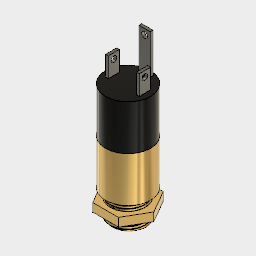
3692 TRS Jack (Autodesk Fusion 360 design; units mm, degrees)
Autodesk Fusion 360 part; units mm, degrees
sketch "Sketch1" plane through (0, 0, 0) normal (0, 0, 1) x (1, 0, 0)
  circle A0 centre (0, 0) radius 3
  dimension "d1" = 6
  measures "d1" diameter of A0
extrude "Extrude1" add sketch "Sketch1" along normal blind 4.6 makes body 1
sketch "Sketch2" plane through (0, 0, 4.6) normal (0, 0, 1) x (-1, 0, 0)
  circle A0 centre (0, 0) radius 3
  circle A1 centre (0, 0) radius 4
  dimension "d4" = 8
  measures "d4" diameter of A1
extrude "Extrude2" add sketch "Sketch2" along normal blind 8 contours A0 | A1 bodies 1
sketch "Sketch3" plane through (0, 0, 4.6) normal (0, 0, -1) x (1, 0, 0)
  circle A0 centre (0, 0) radius 4
  circle A1 centre (0, 0) radius 3
  line L0 (4.6, 0) -> (2.3, 3.9837)
  line L1 (2.3, 3.9837) -> (-2.3, 3.9837)
  line L2 (-2.3, 3.9837) -> (-4.6, 0)
  line L3 (-4.6, 0) -> (-2.3, -3.9837)
  line L4 (-2.3, -3.9837) -> (2.3, -3.9837)
  line L5 (2.3, -3.9837) -> (4.6, 0)
  dimension "d24" = 4.6
  measures "d24" distance of L0.start A0.centre
extrude "Extrude3" add sketch "Sketch3" along normal blind 1.5 from surface at 1.5 separate body contours A0 L0 L1 L2 L3 L4 L5 | A0 L0 L5 | A0 L0 L1 | A0 L4 L5 | A0 L1 L2 | A0 L3 L4 | A0 L2 L3 makes body 2
sketch "Sketch4" plane through (0, 0, 12.6) normal (0, 0, 1) x (-1, 0, 0)
  circle A0 centre (0, 0) radius 4
extrude "Extrude4" add sketch "Sketch4" along normal blind 8 separate body makes body 3
sketch "Sketch5" plane through (0, 0, 20.6) normal (0, 0, 1) x (-1, 0, 0)
  circle A0 centre (0, 0) radius 4
  line L0 (-2.5, -1) -> (-3, -1)
  line L1 (-3, -1) -> (-3, 1)
  line L2 (-3, 1) -> (-2.5, 1)
  line L3 (-2.5, 1) -> (-2.5, -1)
  line L4 (2.5, -1) -> (3, -1)
  line L5 (3, -1) -> (3, 1)
  line L6 (3, 1) -> (2.5, 1)
  line L7 (2.5, 1) -> (2.5, -1)
  line L8 (0, 0) -> (-5, 0) construction
  line L9 (0, 0) -> (5, 0) construction
  line L10 (1, -2.95) -> (-1, -2.95)
  line L11 (-1, -2.95) -> (-1, -3.45)
  line L12 (-1, -3.45) -> (1, -3.45)
  line L13 (1, -3.45) -> (1, -2.95)
  line L14 (1, -2.95) -> (-1, -3.45) construction
  line L15 (-1, -2.95) -> (1, -3.45) construction
  point P0 (0, -3.2)
  dimension "d14" = 0.5
  dimension "d15" = 2
  dimension "d16" = 2
  dimension "d17" = 0.5
  dimension "d27" = 2
  dimension "d28" = 0.5
  dimension "d29" = 3.2
  measures "d14" distance of L0.start L0.end
  measures "d15" distance of L0.start L2.end
  measures "d16" distance of L4.start L6.end
  measures "d17" distance of L4.start L4.end
  measures "d27" distance of L11.end L12.end
  measures "d28" distance of L10.end L11.end
  measures "d29" distance of A0.centre P0
extrude "Extrude5" add sketch "Sketch5" along normal blind 7 separate body contours L10 L11 L12 L13 makes body 4
extrude "Extrude6" add sketch "Sketch5" along normal blind 3.5 separate body contours L0 L1 L2 L3 | L4 L5 L6 L7 makes body 5 at (-2.5, -0.3333, 21.7667) makes body 6 at (3, 0.3333, 21.7667)
sketch "Sketch6" plane through (-3, 0, 0) normal (-1, 0, 0) x (0, -1, 0)
  line L0 (-1, 20.6) -> (1, 20.6)
  line L1 (1, 20.6) -> (1, 24.1)
  line L2 (1, 24.1) -> (-1, 24.1)
  line L3 (-1, 24.1) -> (-1, 20.6)
  circle A0 centre (0, 23.1) radius 0.5
  dimension "d30" = 1
  dimension "d31" = 1
  measures "d30" diameter of A0
  measures "d31" distance of L2 A0.centre
extrude "Extrude7" cut sketch "Sketch6" against normal up to surface (6 mm away) contours A0 bodies 5 6
sketch "Sketch7" plane through (0, 3.45, 0) normal (0, 1, 0) x (-1, 0, 0)
  line L0 (-1, 20.6) -> (1, 20.6)
  line L1 (1, 20.6) -> (1, 27.6)
  line L2 (1, 27.6) -> (-1, 27.6)
  line L3 (-1, 27.6) -> (-1, 20.6)
  circle A0 centre (0, 26.6) radius 0.5
  dimension "d34" = 1
  dimension "d35" = 1
  measures "d34" diameter of A0
  measures "d35" distance of L2 A0.centre
extrude "Extrude8" cut sketch "Sketch7" against normal up to surface (0.5 mm away) contours A0 bodies 4
sketch "Sketch8" plane through (0, 0, 0) normal (0, 0, -1) x (1, 0, 0)
  circle A0 centre (0, 0) radius 3
  circle A1 centre (0, 0) radius 2.2
  dimension "d38" = 0.8
extrude "Extrude9" cut sketch "Sketch8" against normal blind 6 contours A1 bodies 1
thread "Thread1" "ANSI Unified Screw Threads 0.25 1/4-56 UNS 2A" major diameter 6.2789 minor diameter 5.7912 pitch 0.4536 angle 60 modelled right hand crest width 0.0567 on face at (2.9851, -0.2987, 1.5333) crest through (3.1394, 0, -0.0283) on bodies 1
named bodies: "plug", "body", "sleve", "tip (1)", "ring", "hex nut"
